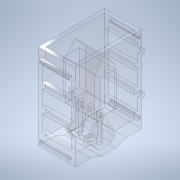
# Autodesk Inventor part: Contenedor
Saved by Autodesk Inventor 2021 (Build 250183000, 183)
## iProperties
Created: 2021-06-28
Part Number: Contenedor
Material: Plástico PBT
Document SubType Name: Modeling
Designer: artur
Density: 1.31 g/cm^3
Appearance: Transparente - Azul pizarra
Mass: 13300.6 g
Surface Area: 10980.8 cm^2
Volume: 10153.1 cm^3
Author: artur
Autodesk Inventor part; units mm, degrees
ref_plane "YZ Plane" through (0, 0, 0) normal (1, 0, 0) x (0, 1, 0)
sketch "Boceto1" plane through (0, 0, 0) normal (0, 0, 1) x (1, 0, 0)
  line L0 (0, 0) -> (100, 0)
  line L1 (0, 300) -> (0, 100)
  line L2 (0, 0) -> (101, 0)
  line L3 (101, 0) -> (101, 400)
  line L4 (101, 400) -> (0, 400)
  line L5 (0, 300) -> (0, 100)
  line L6 (0, 0) -> (89.446919, 0) construction
  line L7 (89.446919, 0) -> (89.446919, 328.576427) construction
  line L8 (89.446919, 328.576427) -> (0, 328.576427) construction
  line L9 (0, 328.576427) -> (0, 0) construction
  line L10 (0, 300) -> (-100, 300) construction
  line L11 (-100, 300) -> (-100, 100) construction
  line L12 (-100, 100) -> (0, 100) construction
  line L13 (0, 100) -> (0, 300) construction
  line L14 (0, 300) -> (-100, 300)
  line L15 (-100, 300) -> (-100, 100)
  line L16 (-100, 100) -> (0, 100)
  line L17 (0, 100) -> (0, 300)
  line L18 (-100, 0) -> (-201, 0)
  line L19 (-201, 0) -> (-201, 400)
  line L20 (-201, 400) -> (-100, 400)
  line L21 (-100, 300) -> (-100, 100)
  line L22 (-100, 400) -> (0, 400)
  line L23 (-90, 115) -> (-10, 115)
  line L24 (-10, 115) -> (-10, 290)
  line L25 (-10, 290) -> (-90, 290)
  line L26 (-90, 290) -> (-90, 115)
  line L27 (121, 400) -> (121, -40.11496)
  line L28 (-221, -40.11496) -> (-221, 400)
  line L29 (-221, 400) -> (-201, 400)
  line L30 (101, 400) -> (121, 400)
  line L31 (-100, 100) -> (-100, 0) construction
  line L32 (-50, -10.001697) -> (-50, -88.070019) construction
  arc A0 (-86.631712, -60.254778) -> (-221, -40.11496) centre (-181.699102, -236.215545) ccw
  arc A1 (121, -40.11496) -> (-13.368288, -60.254778) centre (81.699102, -236.215545) ccw
  line L33 (-100, 0) -> (-100, -21.753366)
  line L34 (-100, 400) -> (-100, 300) construction
  line L35 (-36.354168, -10.586421) -> (-36.354168, -60.254778) construction
  line L36 (-36.354168, -60.254778) -> (-13.368288, -60.254778)
  line L37 (-36.354168, -60.254778) -> (-86.631712, -60.254778)
  line L38 (-80.7634, -42.796987) -> (-50, -42.796987)
  line L39 (-80.7634, -42.796987) -> (-100, -21.753366)
  line L40 (0, 0) -> (0, -21.753366)
  line L41 (-19.2366, -42.796987) -> (-50, -42.796987)
  line L42 (-19.2366, -42.796987) -> (0, -21.753366)
  line L43 (121, -40.11496) -> (-221, -40.11496)
  point P0 (-22.932327, -60.254778)
  point P1 (-67.209235, -60.254778)
  point P2 (-1, -10.708427)
  point P3 (-10, -48.313107)
  point P4 (-50, 290)
  point P5 (-90, 250)
  point P6 (42.398205, -40.11496)
  point P7 (-142.398205, -40.11496)
  dimension "d2" = 101
  dimension "d9" = 101
  dimension "d11" = 400
  dimension "d12" = 100
  dimension "d13" = 200
  dimension "d14" = 100
  dimension "d15" = 10
  dimension "d16" = 15
  dimension "d17" = 10
  dimension "d18" = 10
  dimension "d19" = 20
  dimension "d27" = 302
  dimension "d31" = 200
  dimension "d36" = 20
  dimension "d129" = 205
  dimension "d225" = 100
  dimension "d226" = 100
  constraints: 88 end point, 15 parallel, 13 horizontal, 8 point on line, 7 perpendicular, 4 point on circle, 2 centre point, 2 symmetric about line, 2 vertical, 1 collinear, 1 midpoint, 1 other
  measures "d2" distance of L3.end L4.end
  measures "d9" distance of L19.end L20.end
  measures "d11" distance of L18.end L19.end
  measures "d12" distance of L20.end L4.end
  measures "d13" distance of L10.end L11.end
  measures "d14" distance of L11.end L1.end
  measures "d15" distance between parallel lines of L25 L10
  measures "d16" distance between parallel lines of L23 L12
  measures "d17" distance between parallel lines of L1 L24
  measures "d18" distance between parallel lines of L26 L11
  measures "d19" distance between parallel lines of L19 L28
  measures "d27" distance between parallel lines of L3 L19
  measures "d31" radius of A1
  measures "d36" distance between parallel lines of L27 L3
  measures "d129" distance from line of L42 A1.centre
  measures "d225" distance between parallel lines of L18 L12
  measures "d226" distance between parallel lines of L12 L2
extrude "Extrusión1" add sketch "Boceto1" against normal blind 151 contours L0 L2 L3 L30 L27 A1 L43 L42 L40 | L43 A1 L36 L37 A0 L39 L38 L41 L42 | A1 L43 | L43 A0 L28 L29 L19 L18 L33 L39 | L43 A0 | L1 L16 L15 L14
sketch "Boceto2" plane through (0, 0, 0) normal (0, 0, 1) x (1, 0, 0)
  line L0 (-221, 400) -> (-221, -40.11496)
  line L1 (121, -40.11496) -> (121, 400)
  arc A0 (121, -40.11496) -> (-13.368288, -60.254778) centre (81.699102, -236.215545) ccw
  arc A1 (-86.631712, -60.254778) -> (-221, -40.11496) centre (-181.699102, -236.215545) ccw
  line L2 (-86.631712, -74.888772) -> (-13.368288, -74.888772)
  line L3 (-221, 400) -> (121, 400)
  line L4 (-201, 0) -> (-201, 400)
  line L5 (-90, 115) -> (-90, 290)
  line L6 (-90, 290) -> (-10, 290)
  line L7 (-10, 115) -> (-90, 115)
  line L8 (-10, 290) -> (-10, 115)
  line L9 (42.398205, -40.11496) -> (121, -40.11496)
  line L10 (-221, -40.11496) -> (-142.398205, -40.11496)
  point P0 (0, 0)
  constraints: 2 end point, 1 perpendicular
sketch "Boceto2 outline for Extrusión2" plane through (0, 0, 0) normal (0, 0, 1) x (1, 0, 0)
  line L0 (-221, 400) -> (-221, -40.11496)
  line L1 (-221, -40.11496) -> (-142.398205, -40.11496)
  arc A0 (-142.398205, -40.11496) -> (-86.631712, -60.254778) centre (-181.699102, -236.215545) cw
  line L2 (-86.631712, -60.254778) -> (-13.368288, -60.254778)
  arc A1 (-13.368288, -60.254778) -> (42.398205, -40.11496) centre (81.699102, -236.215545) cw
  line L3 (42.398205, -40.11496) -> (121, -40.11496)
  line L4 (121, -40.11496) -> (121, 400)
  line L5 (121, 400) -> (-221, 400)
  line L6 (-90, 115) -> (-90, 290)
  line L7 (-90, 290) -> (-10, 290)
  line L8 (-10, 290) -> (-10, 115)
  line L9 (-10, 115) -> (-90, 115)
extrude "Extrusión2" add sketch "Boceto2 outline for Extrusión2" along normal blind 20
ref_plane "Plano de trabajo4" through (0, 0, -75.5) normal (0, 0, 1) x (1, 0, 0)
mirror "Simetría2" about plane through (0, 0, -75.5) normal (0, 0, 1) of "Extrusión2"
sketch "Boceto11" plane through (121, -40.11496, 20) normal (1, 0, 0) x (0, 0, -1)
  line L0 (0, 155.11496) -> (0, 330.11496)
  line L1 (20, 40.11496) -> (171, 40.11496)
  line L2 (171, 18.361594) -> (171, 40.11496)
  line L3 (20, 40.11496) -> (171, 40.11496)
  line L4 (171, 40.11496) -> (171, 25.11496)
  line L5 (171, 25.11496) -> (20, 25.11496)
  line L6 (20, 25.11496) -> (20, 40.11496)
  line L7 (171, 440.11496) -> (171, 40.11496)
  line L8 (20, 400.11496) -> (171, 400.11496)
  line L9 (171, 400.11496) -> (171, 385.11496)
  line L10 (171, 385.11496) -> (20, 385.11496)
  line L11 (20, 385.11496) -> (20, 400.11496)
  line L12 (191, 440.11496) -> (0, 440.11496)
  line L13 (20, 40.11496) -> (20, 440.11496)
  line L14 (0, 440.11496) -> (0, 0)
  line L15 (20, 350.11496) -> (0, 350.11496)
  line L16 (0, 350.11496) -> (0, 330.11496)
  line L17 (0, 330.11496) -> (20, 330.11496)
  line L18 (20, 330.11496) -> (20, 350.11496)
  line L19 (191, 330.11496) -> (0, 330.11496)
  line L20 (0, 135.11496) -> (20, 135.11496)
  line L21 (20, 135.11496) -> (20, 155.11496)
  line L22 (20, 155.11496) -> (0, 155.11496)
  line L23 (0, 155.11496) -> (0, 135.11496)
  line L24 (191, 155.11496) -> (0, 155.11496)
  point P0 (0, 155.11496)
  point P1 (20, 135.11496)
  point P2 (20, 330.11496)
  point P3 (0, 350.11496)
  dimension "d227" = 15
  dimension "d228" = 15
  dimension "d229" = 40
  dimension "d230" = 20
  dimension "d231" = 0
  dimension "d232" = 20
  dimension "d233" = 0
  constraints: 32 end point, 8 parallel, 6 point on line, 4 horizontal, 4 perpendicular
  measures "d227" distance of L3.end L4.end
  measures "d228" distance of L8.end L9.end
  measures "d229" distance between parallel lines of L8 L12
  measures "d230" distance between parallel lines of L15 L17
  measures "d231" distance between parallel lines of L17 L19
  measures "d232" distance between parallel lines of L22 L20
  measures "d233" distance between parallel lines of L24 L22
extrude "Extrusión8" add sketch "Boceto11" along normal blind 13 contours L22 L13 L20 L14 | L14 L15 L13 L17 | L1 L2 L5 L6 | L11 L8 L7 L10
sketch "Boceto17" plane through (0, 0, 20) normal (0, 0, 1) x (1, 0, 0)
  line L0 (-100, 300) -> (-100, 100)
  line L1 (-100, 300) -> (-50, 362.44998)
  line L2 (-50, 362.44998) -> (0, 300)
  line L3 (0, 300) -> (-100, 300)
  point P0 (0, 0)
  dimension "d132" = 80
  dimension "d133" = 80
  constraints: 4 end point
  measures "d132" distance of L1.end L2.end
  measures "d133" distance of L0.start L1.end
extrude "Extrusión14" add sketch "Boceto17" against normal up to surface (191 mm away)
sketch "Boceto20" plane through (-86.631712, -60.254778, 20) normal (0, -1, 0) x (1, 0, 0)
  line L0 (36.631712, -20) -> (36.631712, -171)
  circle A0 centre (36.631712, -95.5) radius 25
  point P0 (86.631712, -20)
  dimension "d161" = 50
  constraints: 1 centre point, 1 midpoint
  measures "d161" diameter of A0
extrude "Extrusión16" cut sketch "Boceto20" against normal blind 50
sketch "Boceto24" plane through (121, -40.11496, -171) normal (1, 0, 0) x (0, 0, -1)
  line L0 (-171, 70.11496) -> (-20, 70.11496)
  line L1 (-20, 70.11496) -> (-20, 150.11496)
  line L2 (-20, 150.11496) -> (-171, 150.11496)
  line L3 (-171, 150.11496) -> (-171, 70.11496)
  line L4 (-171, 440.11496) -> (-171, 40.11496)
  line L5 (-20, 40.11496) -> (-20, 440.11496)
  line L6 (-171, 260.11496) -> (-171, 180.11496)
  line L7 (-20, 260.11496) -> (-171, 260.11496)
  line L8 (-171, 180.11496) -> (-20, 180.11496)
  line L9 (-20, 180.11496) -> (-20, 260.11496)
  line L10 (-171, 370.11496) -> (-171, 290.11496)
  line L11 (-20, 370.11496) -> (-171, 370.11496)
  line L12 (-171, 290.11496) -> (-20, 290.11496)
  line L13 (-20, 290.11496) -> (-20, 370.11496)
  line L14 (-40, 20) -> (-191, 20)
  line L15 (-171, 40.11496) -> (-20, 40.11496)
  point P0 (-20, 180.11496)
  point P1 (-20, 260.11496)
  point P2 (-20, 290.11496)
  point P3 (-20, 370.11496)
  dimension "d210" = 0
  dimension "d211" = 0
  dimension "d213" = 80
  dimension "d216" = 110
  dimension "d242" = 30
  constraints: 24 end point, 2 parallel, 1 horizontal, 1 perpendicular, 1 vertical, 16 other
  measures "d210" distance between parallel lines of L3 L4
  measures "d211" distance between parallel lines of L1 L5
  measures "d213" distance of L0.end L1.end
  measures "d216" distance of L2.end L6.start
  measures "d242" distance between parallel lines of L0 L15
extrude "Extrusión19" cut sketch "Boceto24" against normal blind 90.5 contours L3 L2 L1 L0 | L4 L7 L5 L8 | L4 L11 L5 L12
ref_plane "Plano de trabajo8" through (-50, -40.11496, -171) normal (1, 0, 0) x (0, 0, -1)
mirror "Simetría11" about plane through (-50, -40.11496, -171) normal (1, 0, 0) of "Extrusión19"
sketch "Boceto19" plane through (0, 0, -75.5) normal (0, 0, 1) x (1, 0, 0)
  line L0 (101, 0) -> (0, 0)
  line L1 (-100, 100) -> (0, 100)
  line L2 (5.035969, -3.185244) -> (-50, 106.67627)
  line L3 (-50, 106.67627) -> (-42.05592, 113.144973)
  line L4 (-50, 106.67627) -> (-50, 46.415991) construction
  line L5 (-42.05592, 113.144973) -> (28.159909, -27.018223)
  line L6 (28.159909, -27.018223) -> (19.219064, -31.497207)
  line L7 (19.219064, -31.497207) -> (5.035969, -3.185244)
  line L8 (0, 100) -> (0, 300)
  point P0 (8.947701, 0)
  point P1 (-35.470845, 100)
  point P2 (-46.655471, 100)
  point P3 (3.440296, 0)
  point P4 (14.624923, 0)
  dimension "d185" = 50
  dimension "d186" = 100
  dimension "d187" = 10
  constraints: 12 end point, 2 perpendicular, 1 parallel, 1 point on line, 1 vertical
  measures "d185" distance from line of L8 L2.end
  measures "d186" distance of L1.start L1.end
  measures "d187" distance between parallel lines of L5 L2
sketch "Boceto19 outline for Revolución1" plane through (0, 0, -75.5) normal (0, 0, 1) x (1, 0, 0)
  line L0 (-42.05592, 113.144973) -> (-50, 106.67627)
  line L1 (-50, 106.67627) -> (19.219064, -31.497207)
  line L2 (19.219064, -31.497207) -> (28.159909, -27.018223)
  line L3 (28.159909, -27.018223) -> (-42.05592, 113.144973)
revolve "Revolución1" add sketch "Boceto19 outline for Revolución1" angle 360 about axis through (5.035969, -3.185244, -75.5) along (-0.4478985, 0.8940844, 0)
pattern_linear "Patrón rectangular3" count 2 spacing 50 along (0, 0, -1) count 2 spacing 50 along (0, 0, 1) of "Revolución1" second direction both ways yes
sketch "Boceto25" plane through (121, 345, -151) normal (0, -1, 0) x (1, 0, 0)
  line L0 (0, 151) -> (13, 151) projected
  line L1 (13, 151) -> (0, 151)
  line L2 (0, 0) -> (13, 0) projected
  line L3 (0, 151) -> (10, 151)
  line L4 (10, 151) -> (10, 0)
  line L5 (10, 0) -> (0, 0)
  line L6 (0, 0) -> (0, 151)
  point P0 (-121, 151)
  point P1 (0, 0)
  dimension "d234" = 13
  dimension "d235" = 10
  constraints: 10 end point, 2 parallel, 2 point on line, 1 horizontal, 1 perpendicular
  measures "d234" distance of L0.end L1.end
  measures "d235" distance of L4.end L5.end
extrude "Extrusión20" cut sketch "Boceto25" against normal blind 5
sketch "Boceto26" plane through (121, 0, 0) normal (0, 1, 0) x (1, 0, 0)
  line L0 (13, 0) -> (13, 151) projected
  line L1 (13, 0) -> (0, 0)
  line L2 (0, 0) -> (13, 0) projected
  line L3 (0, 0) -> (10, 0)
  line L4 (10, 0) -> (10, 151)
  line L5 (10, 151) -> (0, 151)
  line L6 (0, 151) -> (0, 0)
  point P0 (-121, 0)
  point P1 (10, 0)
  dimension "d238" = 13
  dimension "d239" = 10
  constraints: 10 end point, 2 parallel, 1 horizontal, 1 perpendicular, 1 point on line
  measures "d238" distance of L0.start L1.end
  measures "d239" distance of L5.end L4.end
extrude "Extrusión21" cut sketch "Boceto26" against normal blind 5
mirror "Simetría13" about plane through (-50, -40.11496, -171) normal (1, 0, 0) of "Extrusión8", "Extrusión20", "Extrusión21"
mirror "Simetría14" about plane through (-50, -40.11496, -171) normal (1, 0, 0) of "Revolución1", "Patrón rectangular3"
sketch "Boceto27" plane through (-90, 115, 20) normal (0, 1, 0) x (1, 0, 0)
  ellipse E0 centre (43.344529, 95.5) end of major axis (54.529155, 95.5) minor radius 10 (40, 85.95756) -> (40, 105.04244) ccw
  ellipse E1 centre (36.655471, 145.5) end of major axis (25.470845, 145.5) minor radius 10 (40, 155.04244) -> (40, 135.95756) ccw
  ellipse E2 centre (43.344529, 145.5) end of major axis (54.529155, 145.5) minor radius 10 (40, 135.95756) -> (40, 155.04244) ccw
  ellipse E3 centre (36.655471, 45.5) end of major axis (25.470845, 45.5) minor radius 10 (40, 55.04244) -> (40, 35.95756) ccw
  ellipse E4 centre (43.344529, 45.5) end of major axis (54.529155, 45.5) minor radius 10 (40, 35.95756) -> (40, 55.04244) ccw
  point P0 (90, 20)
  constraints: 5 other
extrude "Extrusión22" add sketch "Boceto27" against normal up to surface (175.254778 mm away)
thread "Rosca2" size "M50x4" class "6H" standard "ANSI Metric M Profile" full length
